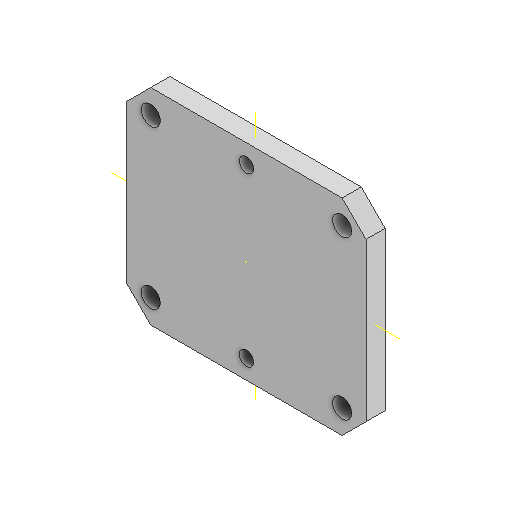
# Autodesk Inventor part: 집게_고정대
Saved by Autodesk Inventor 2027 (Build 310192000, 192)
## iProperties
Created: 2026-09-23
Part Number: 집게_고정대
Material: 일반
Document SubType Name: Modeling
Designer: User
Density: 1 g/cm^3
Appearance: 기본값
Author: User
Autodesk Inventor part; units mm, degrees
ref_plane "YZ 평면_우측면도" through (0, 0, 0) normal (1, 0, 0) x (0, 1, 0)
ref_plane "XZ 평면_평면도" through (0, 0, 0) normal (0, 1, 0) x (-1, 0, 0)
ref_plane "XY 평면_정면도" through (0, 0, 0) normal (0, 0, 1) x (1, 0, 0)
sketch "스케치1" plane through (0, 0, 0) normal (0, 0, 1) x (1, 0, 0)
  line L0 (20, -21.5) -> (-20, -21.5)
  line L1 (-25, -16.5) -> (-25, 16.5)
  line L2 (-20, 21.5) -> (20, 21.5)
  line L3 (25, 16.5) -> (25, -16.5)
  line L4 (25, -21.5) -> (-25, 21.5) construction
  line L5 (-25, -21.5) -> (25, 21.5) construction
  line L6 (0, 21.5) -> (0, -21.5) construction
  line L7 (-25, 17.5) -> (25, 17.5) construction
  circle A0 centre (0, 17.5) radius 1.5
  line L8 (-25, -17.5) -> (25, -17.5) construction
  circle A1 centre (0, -17.5) radius 1.5
  line L9 (-25, -16.5) -> (25, -16.5) construction
  line L10 (-25, 16.5) -> (25, 16.5) construction
  line L11 (-20, 21.5) -> (-20, -21.5) construction
  line L12 (20, 21.5) -> (20, -21.5) construction
  circle A2 centre (-20, 16.5) radius 2
  circle A3 centre (-20, -16.5) radius 2
  circle A4 centre (20, 16.5) radius 2
  circle A5 centre (20, -16.5) radius 2
  line L13 (-20, 21.5) -> (-25, 16.5)
  line L14 (-25, -16.5) -> (-20, -21.5)
  line L15 (20, 21.5) -> (25, 16.5)
  line L16 (25, -16.5) -> (20, -21.5)
  point P0 (0, 0)
  dimension "d0" = 50
  dimension "d1" = 43
  dimension "d2" = 4
  dimension "d3" = 3
  dimension "d4" = 4
  dimension "d5" = 3
  dimension "d7" = 5
  dimension "d8" = 5
  dimension "d9" = 5
  dimension "d10" = 5
  dimension "d11" = 4
  dimension "d12" = 4
  dimension "d13" = 4
  dimension "d14" = 4
  dimension "d15" = 5
  dimension "d16" = 5
  dimension "d17" = 5
  dimension "d18" = 5
  dimension "d19" = 5
  dimension "d20" = 5
  dimension "d21" = 5
  dimension "d22" = 5
  constraints: 34 end point, 24 point on line, 6 centre point, 6 midpoint, 4 parallel, 3 perpendicular, 2 horizontal
  measures "d0" distance of L4.end L5.end
  measures "d1" distance of L5.start L4.end
  measures "d2" distance between parallel lines of L7 L2
  measures "d3" diameter of A0
  measures "d4" distance between parallel lines of L0 L8
  measures "d5" diameter of A1
  measures "d7" distance between parallel lines of L0 L9
  measures "d8" distance between parallel lines of L10 L2
  measures "d9" distance between parallel lines of L1 L11
  measures "d10" distance between parallel lines of L3 L12
  measures "d11" diameter of A2
  measures "d12" diameter of A3
  measures "d13" diameter of A4
  measures "d14" diameter of A5
  measures "d15" distance of L2.start L4.end
  measures "d16" distance of L1.end L4.end
  measures "d17" distance of L1.start L5.start
  measures "d18" distance of L0.end L5.start
  measures "d19" distance of L2.end L5.end
  measures "d20" distance of L3.start L5.end
  measures "d21" distance of L3.end L4.start
  measures "d22" distance of L0.start L4.start
extrude "돌출1" add sketch "스케치1" along normal mid plane 4
equation "\"d16\" = d15"
equation "\"d17\" = d15"
equation "\"d18\" = d17"
equation "\"d19\" = d15"
equation "\"d20\" = d19"
equation "\"d21\" = d15"
equation "\"d22\" = d21"
